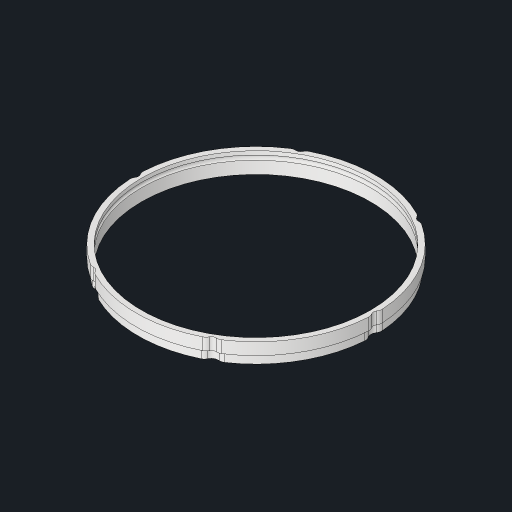
# Autodesk Inventor part: Ring Driving Track
Saved by Autodesk Inventor 2023.2 (Build 272271030, 271C)
## iProperties
Created: 2024-02-21
Part Number: Ring Driving Track
Material: Generic
Document SubType Name: Modeling
Designer: robpl
Density: 1 g/cm^3
Appearance: Default
Author: robpl
Autodesk Inventor part; units mm, degrees
ref_plane "YZ Plane" through (0, 0, 0) normal (1, 0, 0) x (0, 1, 0)
ref_plane "XZ Plane" through (0, 0, 0) normal (0, 1, 0) x (-1, 0, 0)
ref_plane "XY Plane" through (0, 0, 0) normal (0, 0, 1) x (1, 0, 0)
sketch "Sketch1" plane through (0, 0, 0) normal (0, 0, 1) x (1, 0, 0)
  line L0 (-67, 0) -> (-70, 0)
  line L1 (-70, 0) -> (-70, 7)
  line L2 (-70, 7) -> (-67, 7)
  line L3 (-67, 7) -> (-67, 0)
  line L4 (-67, 0) -> (-69, 0)
  line L5 (-69, 0) -> (-69, -5)
  line L6 (-69, -5) -> (-67, -5)
  line L7 (-67, -5) -> (-67, 0)
  line L8 (0, -7.4) -> (0, 9.4) projected
  circle A0 centre (-65.5, 3.5) radius 2
  point P0 (0, 0)
  point P1 (-69, 0)
  point P2 (-67.5, 3.5)
  point P3 (-70, 3.5)
  point P4 (-67, 2.1771)
  point P5 (-67, 4.8229)
  dimension "d27" = 4
  dimension "d0" = 5
  dimension "d1" = 69
  dimension "d4" = 7
  dimension "d7" = 67
  dimension "d28" = 67.5
  dimension "d29" = 1
  constraints: 16 end point, 4 parallel, 2 horizontal, 2 horizontal alignment, 2 perpendicular, 1 midpoint, 1 point on line, 3 other
  measures "d0" distance of L6.end L0.start
  measures "d1" distance from line of point (0, 0) L5
  measures "d4" distance of L2.end L0.start
  measures "d7" distance from line of point (0, 0) L7
  measures "d28" horizontal distance of point (0, 0) point (-67.5, 3.5)
  measures "d29" distance between parallel lines of L5 L1
revolve "Revolution1" add sketch "Sketch1" angle 360 about axis through (0, -10, 0) along (0, 1, 0) contours L7 L6 L5 L0 | L0 L1 L2 L3 A0
sketch "Sketch2" plane through (0, 7, 0) normal (0, 1, 0) x (1, 0, 0)
  circle A0 centre (-71.25, 0) radius 2.55
  point P0 (0, 0)
  dimension "d16" = 5.1
  dimension "d17" = 71.25
  constraints: 1 centre point, 1 horizontal alignment
  measures "d16" diameter of A0
  measures "d17" distance of point (0, 0) A0.centre
extrude "Extrusion1" cut sketch "Sketch2" against normal through all
sketch "Sketch3" plane through (0, -5, 0) normal (0, -1, 0) x (1, 0, 0)
  arc A0 (-68.9899, -1.1809) -> (-68.9899, 1.1809) centre (-71.25, 0) ccw projected
  circle A1 centre (-71.25, 0) radius 4
  point P0 (0, 0)
  dimension "d20" = 8
  constraints: 1 centre point, 1 coincident
  measures "d20" diameter of A1
extrude "Extrusion2" cut sketch "Sketch3" against normal up to surface (5 mm away)
fillet "Fillet1" radius 4 4 edges at (-68.9232, -2.5, -3.2536) (-68.9232, -2.5, 3.2536) (-69.9653, 3.5, -2.2028) (-69.9653, 3.5, 2.2028)
pattern_circular "Circular Pattern1" count 6 over 360 about axis through (0, 3.5, 0) along (0, 1, 0) of "Fillet1", "Extrusion1", "Extrusion2"
body "Solid1"
